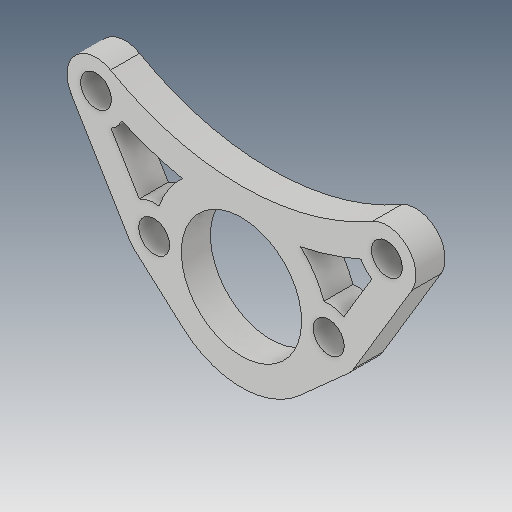
# Autodesk Inventor part: EncoderMount
Saved by Autodesk Inventor 2019.4 (Build 234330000, 330)
## iProperties
Created: 2019-06-28
Part Number: EncoderMount
Material: Generic
Document SubType Name: Modeling
Designer: AzLIer
Density: 1 g/cm^3
Appearance: Default
Author: AzLIer
Autodesk Inventor part; units mm, degrees
ref_plane "YZ Plane" through (0, 0, 0) normal (1, 0, 0) x (0, 1, 0)
ref_plane "XZ Plane" through (0, 0, 0) normal (0, 1, 0) x (-1, 0, 0)
ref_plane "XY Plane" through (0, 0, 0) normal (0, 0, 1) x (1, 0, 0)
sketch "スケッチ1" plane through (0, 0, 0) normal (0, 0, 1) x (1, 0, 0)
  circle A0 centre (0, 0) radius 6.2
  line L0 (-9, 0) -> (9, 0) construction
  circle A1 centre (9, 0) radius 1.6
  circle A2 centre (-9, 0) radius 1.6
  line L1 (15, 10) -> (-15, 10) construction
  circle A3 centre (15, 10) radius 1.6
  circle A4 centre (-15, 10) radius 1.6
  arc A5 (-6.1356, 0.8916) -> (-6.1356, -0.8916) centre (-9, 0) ccw
  arc A6 (6.1356, -0.8916) -> (6.1356, 0.8916) centre (9, 0) ccw
  line L2 (17.5725, 8.4565) -> (11.5725, -1.5435)
  line L3 (11, -2.2361) -> (6, -6.7082)
  line L4 (-6, -6.7082) -> (-11, -2.2361)
  line L5 (-11.5725, -1.5435) -> (-17.5725, 8.4565)
  arc A7 (-13.5062, 12.6017) -> (13.5062, 12.6017) centre (0, 36.125) ccw
  arc A8 (-8.5, -2.958) -> (8.5, -2.958) centre (0, 0) ccw
  arc A9 (-12.3272, 8.6376) -> (-6.0941, 6.6228) centre (0, 36.125) ccw
  arc A10 (6.0941, 6.6228) -> (12.3272, 8.6376) centre (0, 36.125) ccw
  line L6 (-10.5435, 2.5725) -> (-13.4565, 7.4275)
  line L7 (13.4565, 7.4275) -> (10.5435, 2.5725)
  arc A11 (8.5, 2.958) -> (6.0941, 6.6228) centre (0, 0) ccw
  arc A12 (-6.0941, 6.6228) -> (-8.5, 2.958) centre (0, 0) ccw
  arc A13 (-13.5062, 12.6017) -> (-17.5725, 8.4565) centre (-15, 10) ccw
  arc A14 (-13.4565, 7.4275) -> (-12.3272, 8.6376) centre (-15, 10) ccw
  arc A15 (17.5725, 8.4565) -> (13.5062, 12.6017) centre (15, 10) ccw
  arc A16 (12.3272, 8.6376) -> (13.4565, 7.4275) centre (15, 10) ccw
  point P0 (0, 10)
  dimension "d0" = 12.4
  dimension "d1" = 18
  dimension "d2" = 3.2
  dimension "d3" = 3.2
  dimension "d4" = 3.2
  dimension "d5" = 3.2
  dimension "d6" = 10
  dimension "d7" = 30
  dimension "d10" = 6
  dimension "d11" = 6
  dimension "d13" = 9
  dimension "d15" = 3
  dimension "d18" = 3
  dimension "d20" = 3
  dimension "d21" = 3
  constraints: 40 point on circle, 17 centre point, 16 end point, 13 tangent, 10 coincident, 4 equal radius, 2 horizontal, 2 midpoint, 2 parallel, 1 concentric, 1 vertical alignment
  measures "d0" diameter of A0
  measures "d1" distance of L0.start L0.end
  measures "d2" diameter of A1
  measures "d3" diameter of A2
  measures "d4" diameter of A3
  measures "d5" diameter of A4
  measures "d6" distance from line of point (0, 0) L1
  measures "d7" distance of L1.start L1.end
  measures "d10" diameter of A5
  measures "d11" diameter of A6
  measures "d13" radius of A8
  measures "d15" radial gap between concentric circles of A10 A7
  measures "d18" distance between parallel lines of L2 L7
  measures "d20" distance between parallel lines of L5 L6
  measures "d21" radius of A13
extrude "押し出し1" add sketch "スケッチ1" along normal blind 3 contours A0 A6 | A0 A5 A12 A9 A14 L6 L5 A13 A7 A15 L2 A6 L7 A16 A10 A11 | A6 A8 A5 A0 | A0 A5 | A6 L3 A8 | A8 L4 A5
